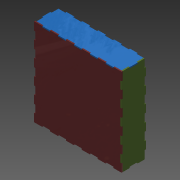
# Autodesk Inventor part: wordClock
Saved by Autodesk Inventor 2015 (Build 190159000, 159)
## iProperties
Created: 2015-02-10
Part Number: wordClock
Material: Generic
Document SubType Name: Modeling
Designer: Iain
Density: 1 g/cm^3
Appearance: Default
Author: Iain
Autodesk Inventor part; units mm, degrees
ref_plane "YZ Plane" through (0, 0, 0) normal (1, 0, 0) x (0, 1, 0)
ref_plane "XZ Plane" through (0, 0, 0) normal (0, 1, 0) x (-1, 0, 0)
ref_plane "XY Plane" through (0, 0, 0) normal (0, 0, 1) x (1, 0, 0)
sketch "Sketch1" plane through (0, 0, 0) normal (0, 0, 1) x (1, 0, 0)
  line L0 (-105, 105) -> (105, 105)
  line L1 (105, 105) -> (105, -105)
  line L2 (105, -105) -> (-105, -105)
  line L3 (-105, -105) -> (-105, 105)
  point P0 (0, 0)
  point P1 (0, 105)
  point P2 (-105, 0)
  dimension "FrontFaceBaseWidth" = 210
  dimension "FrontFaceBaseHeight" = 210
  constraints: 8 end point, 2 midpoint, 2 parallel, 1 horizontal, 1 horizontal alignment, 1 perpendicular, 1 vertical alignment
  measures "FrontFaceBaseWidth" distance of L0.start L0.end
  measures "FrontFaceBaseHeight" distance of L2.end L0.start
extrude "FrontFaceBase" add sketch "Sketch1" along normal mid plane 3
sketch "Sketch4" plane through (0, 0, 1.5) normal (0, 0, 1) x (1, 0, 0)
  line L0 (-108, 108) -> (-88, 108)
  line L1 (-88, 108) -> (-88, 105)
  line L2 (-88, 105) -> (-108, 105)
  line L3 (-108, 105) -> (-108, 108)
  point P0 (-105, 105)
  point P1 (0, 0)
  point P2 (-98, 105)
  dimension "d6" = 3
  dimension "FrontFaceTabWidth" = 20
  dimension "d8" = 3
  constraints: 8 end point, 2 parallel, 1 horizontal, 1 horizontal alignment, 1 midpoint, 1 perpendicular
  measures "d6" distance of point (-105, 105) L2.end
  measures "FrontFaceTabWidth" distance of L0.end L0.start
  measures "d8" distance of L1.end L0.end
extrude "Extrusion2" add sketch "Sketch4" against normal blind 3
pattern_linear "FrontTopTabs" count 6 spacing 39.2 along (1, 0, 0) of "Extrusion2"
sketch "Sketch5" plane through (0, 0, 1.5) normal (0, 0, 1) x (1, 0, 0)
  line L0 (-108, -108) -> (-105, -108)
  line L1 (-105, -108) -> (-105, -88)
  line L2 (-105, -88) -> (-108, -88)
  line L3 (-108, -88) -> (-108, -108)
  point P0 (-105, -105)
  point P1 (0, 0)
  point P2 (-105, -98)
  dimension "d14" = 3
  dimension "d15" = 3
  dimension "d16" = 20
  constraints: 8 end point, 2 parallel, 1 horizontal, 1 midpoint, 1 perpendicular, 1 vertical alignment
  measures "d14" distance of point (-105, -105) L0.end
  measures "d15" distance of L0.start L0.end
  measures "d16" distance of L2.end L0.start
extrude "Extrusion3" add sketch "Sketch5" against normal blind 3
pattern_linear "FontLeftTabs" count 6 spacing 39.2 along (0, 1, 0) of "Extrusion3"
mirror "FrontBottomTabs" about plane through (0, 0, 0) normal (0, 1, 0) of "Extrusion2", "FrontTopTabs"
mirror "FontRightTabs" about plane through (0, 0, 0) normal (1, 0, 0) of "Extrusion3", "FontLeftTabs"
sketch "Sketch6" plane through (-9.6, 105, -1.5) normal (0, 1, 0) x (1, 0, 0)
  line L0 (-98.4, -3) -> (117.6, -3)
  line L1 (117.6, -3) -> (117.6, 57)
  line L2 (117.6, 57) -> (-98.4, 57)
  line L3 (-98.4, 57) -> (-98.4, -3)
  line L4 (-59.2, -3) -> (-78.4, -3) projected
  line L5 (-98.4, -3) -> (-98.4, 0) projected
  point P0 (117.6, 27)
  point P1 (9.6, -3)
  point P2 (-68.8, -3)
  point P3 (-98.4, 27)
  point P4 (-98.4, -1.5)
  dimension "d68" = 216
  dimension "d69" = 60
  constraints: 8 end point, 5 midpoint, 2 parallel, 1 horizontal, 1 horizontal alignment, 1 perpendicular, 1 vertical alignment
  measures "d68" distance of L0.start L0.end
  measures "d69" distance of L0.end L1.end
extrude "TopFaceBase" add sketch "Sketch6" along normal blind 3 separate body
sketch "Sketch7" plane through (-9.6, 108, -1.5) normal (0, 1, 0) x (1, 0, 0)
  line L0 (-98.4, -3) -> (117.6, -3) projected
  line L1 (-98.4, 57) -> (-98.4, -3) projected
  line L2 (-98.4, -3) -> (-78.4, -3)
  line L3 (-78.4, -3) -> (-78.4, 0)
  line L4 (-78.4, 0) -> (-98.4, 0)
  line L5 (-98.4, 0) -> (-98.4, -3)
  point P0 (9.6, -1.5)
  point P1 (-98.4, 27)
  point P2 (9.6, -3)
  dimension "d25" = 20
  dimension "TopFaceFrontSlotDepth" = 3
  constraints: 8 end point, 2 midpoint, 2 parallel, 1 horizontal, 1 horizontal alignment, 1 perpendicular, 1 vertical alignment
  measures "d25" distance of L3.end L4.end
  measures "TopFaceFrontSlotDepth" distance of L2.start L4.end
extrude "Extrusion5" cut sketch "Sketch7" against normal blind 3 bodies 2
sketch "Sketch8" plane through (-9.6, 108, -1.5) normal (0, 1, 0) x (1, 0, 0)
  line L0 (117.6, -3) -> (114.6, -3)
  line L1 (114.6, -3) -> (114.6, 17)
  line L2 (114.6, 17) -> (117.6, 17)
  line L3 (117.6, 17) -> (117.6, -3)
  point P0 (9.6, -1.5)
  dimension "TopSideSlotWidth" = 20
  dimension "d33" = 3
  constraints: 8 end point, 2 parallel, 1 horizontal, 1 perpendicular
  measures "TopSideSlotWidth" distance of L0.end L1.end
  measures "d33" distance of L0.start L0.end
extrude "Extrusion6" cut sketch "Sketch8" against normal blind 3 bodies 2
pattern_linear "TopFrontSlots" count 6 spacing 39.2 along (1, 0, 0) of "Extrusion5", "Extrusion2" bodies 2
pattern_linear "TopSideRightSlots" count 2 spacing 40 along (0, 0, -1) of "Extrusion6" bodies 2
ref_plane "Work Plane1" through (-48.8, 108, -28.5) normal (0, 0, 1) x (1, 0, 0)
mirror "TopBackSlots" about plane through (-48.8, 108, -28.5) normal (0, 0, 1) of "Extrusion5", "Extrusion2", "TopFrontSlots" bodies 2
ref_plane "Work Plane2" through (0, 105, -18.5) normal (1, 0, 0) x (0, 0, -1)
mirror "TopSideLeftSlots" about plane through (0, 105, -18.5) normal (1, 0, 0) of "Extrusion6", "TopSideRightSlots" bodies 2
sketch "Sketch12" plane through (108, 105, -18.5) normal (1, 0, 0) x (0, 0, -1)
  line L0 (0, 0) -> (20, 0) projected
  line L1 (-20, 0) -> (40, 0)
  line L2 (40, 0) -> (40, -210)
  line L3 (40, -210) -> (-20, -210)
  line L4 (-20, -210) -> (-20, 0)
  line L5 (-17, -95.4) -> (-17, -114.6) projected
  line L6 (-20, -114.6) -> (-20, -95.4) projected
  point P0 (-18.5, -105)
  point P1 (10, 0)
  point P2 (10, 0)
  point P3 (-20, -105)
  point P4 (-17, -105)
  point P5 (-20, -105)
  dimension "SideFaceBaseHeight" = 210
  dimension "SideFaceBaseDepth" = 60
  constraints: 8 end point, 5 midpoint, 2 coincident, 2 parallel, 1 horizontal, 1 perpendicular
  measures "SideFaceBaseHeight" distance of L3.end L1.start
  measures "SideFaceBaseDepth" distance of L1.start L1.end
extrude "RightFaceBase" add sketch "Sketch12" against normal blind 3 separate body
sketch "Sketch13" plane through (108, 105, -18.5) normal (1, 0, 0) x (0, 0, -1)
  line L0 (-20, 0) -> (40, 0) projected
  line L1 (-20, 3) -> (0, 3)
  line L2 (0, 3) -> (0, 0)
  line L3 (0, 0) -> (-20, 0)
  line L4 (-20, 0) -> (-20, 3)
  line L5 (-20, -114.6) -> (-20, -95.4) projected
  point P0 (-18.5, -105)
  point P1 (-10, 0)
  point P2 (10, 0)
  point P3 (-20, 1.5)
  point P4 (-20, -105)
  dimension "SideFaceTabWidth" = 20
  dimension "SideTopTabDepth" = 3
  constraints: 8 end point, 4 midpoint, 2 parallel, 1 horizontal, 1 horizontal alignment, 1 perpendicular, 1 vertical alignment
  measures "SideFaceTabWidth" distance of L1.start L1.end
  measures "SideTopTabDepth" distance of L3.end L1.start
extrude "Extrusion9" add sketch "Sketch13" against normal blind 3 bodies 3
pattern_linear "SideTopTabs" count 2 spacing 40 along (0, 0, -1) of "Extrusion9" bodies 3
mirror "SideBottomTabs" about plane through (0, 0, 0) normal (0, 1, 0) of "Extrusion9", "SideTopTabs" bodies 3
sketch "Sketch14" plane through (108, 105, -18.5) normal (1, 0, 0) x (0, 0, -1)
  line L0 (-20, 3) -> (-20, -213) projected
  line L1 (-20, 3) -> (0, 3) projected
  line L2 (-20, 3) -> (-17, 3)
  line L3 (-17, 3) -> (-17, -17)
  line L4 (-17, -17) -> (-20, -17)
  line L5 (-20, -17) -> (-20, 3)
  point P0 (-18.5, -105)
  point P1 (-18.5, 3)
  point P2 (-10, 3)
  point P3 (-20, -7)
  point P4 (-20, -105)
  dimension "d61" = 3
  dimension "d62" = 20
  constraints: 8 end point, 4 midpoint, 2 parallel, 1 horizontal, 1 horizontal alignment, 1 perpendicular, 1 vertical alignment
  measures "d61" distance of L2.start L2.end
  measures "d62" distance of L4.end L2.start
extrude "Extrusion10" cut sketch "Sketch14" against normal blind 3 bodies 3
pattern_linear "SideFrontSlots" count 6 spacing 39.2 along (0, -1, 0) of "Extrusion10" bodies 3
ref_plane "Work Plane4" through (105, 29.6, -28.5) normal (0, 0, 1) x (1, 0, 0)
mirror "SideBackSlots" about plane through (105, 29.6, -28.5) normal (0, 0, 1) of "Extrusion10", "SideFrontSlots" bodies 3
ref_plane "Work Plane3" through (0, 0, 0) normal (0, 1, 0) x (-1, 0, 0)
equation "\"FrontFaceBaseWidth\" = ClockWidth - 2 * FrontFaceTabDepth"
equation "\"FrontFaceBaseHeight\" = ClockHeight - 2 * FrontFaceTabDepth"
equation "\"FrontFaceThickness\" = Ply3mm"
equation "\"d6\" = TabDepth"
equation "\"FrontFaceTabWidth\" = TabWidth"
equation "\"d8\" = FrontFaceTabDepth"
equation "\"d9\" = FrontFaceThickness"
equation "\"d14\" = FrontFaceTabDepth"
equation "\"d15\" = FrontFaceTabDepth"
equation "\"d16\" = FrontFaceTabWidth"
equation "\"d17\" = FrontFaceThickness"
equation "\"d68\" = ClockWidth"
equation "\"d69\" = ClockDepth"
equation "\"TopFaceThickness\" = Ply3mm"
equation "\"d25\" = FrontFaceTabWidth"
equation "\"TopFaceFrontSlotDepth\" = FrontFaceThickness"
equation "\"d27\" = TopFaceThickness"
equation "\"d33\" = TabDepth"
equation "\"d34\" = TopFaceThickness"
equation "\"d38\" = FrontFaceTopTabSpacing"
equation "\"SideFaceBaseHeight\" = ClockHeight - 2 * FrontFaceThickness"
equation "\"SideFaceBaseDepth\" = ClockDepth"
equation "\"SideFaceThickness\" = Ply3mm"
equation "\"SideFaceTabWidth\" = TopSideSlotWidth"
equation "\"SideTopTabDepth\" = TopFaceThickness"
equation "\"d56\" = SideFaceThickness"
equation "\"d60\" = TopFaceSlotsSideSpcaing"
equation "\"d61\" = FrontFaceThickness"
equation "\"d62\" = FrontFaceTabWidth"
equation "\"d63\" = SideFaceThickness"
equation "\"d67\" = FrontFaceSideTabSpacing"
equation "\"FrontFaceTabDepth\" = TabDepth"
equation "\"ClockHeight\" = 216"
equation "\"ClockWidth\" = 216"
equation "\"ClockDepth\" = 60"
equation "\"Ply3mm\" = 3"
equation "\"TabDepth\" = Ply3mm"
equation "\"TabWidth\" = 20"
equation "\"FrontFaceTopTabSpacing\" = 39.2"
equation "\"TopFaceSlotsSideSpcaing\" = 40"
equation "\"FrontFaceSideTabSpacing\" = 39.2"
